2020_Simple_v7 (Autodesk Fusion 360 design; units mm, degrees)
Autodesk Fusion 360 part; units mm, degrees
sketch "Sketch1" plane through (0, 0, 0) normal (1, 0, 0) x (0, 1, 0)
  line L0 (4.6363, -9.9678) -> (4.6743, -9.9793) construction
  line L1 (-9.9374, 4.563) -> (-9.9187, 4.5279) construction
  line L2 (8.5, -10) -> (9.5, -10) construction
  line L3 (10, -9.5) -> (10, -8.5) construction
  line L4 (-9.8746, 4.4619) -> (-9.8494, 4.4312) construction
  line L5 (-9.9187, 4.5279) -> (-9.8977, 4.4942) construction
  line L6 (9.9987, -4.7917) -> (9.9948, -4.7522) construction
  line L7 (9.8977, -4.4942) -> (9.8746, -4.4619) construction
  arc A0 (-8.5414, 3.1214) -> (-8.2, 3.2628) centre (-8.4, 3.2628) ccw construction
  line L8 (10, -4.9) -> (9.9987, -4.7917) construction
  line L9 (-3.9, 2.8393) -> (-3.9, 0.1999) construction
  line L10 (-9.8977, 4.4942) -> (-9.8746, 4.4619) construction
  line L11 (-10, 4.8314) -> (-9.9987, 4.7917) construction
  line L12 (-9.8494, 4.4312) -> (-9.8222, 4.4022) construction
  line L13 (8.2, -5.5) -> (6.5607, -5.5) construction
  line L14 (-6.5607, 5.5) -> (-3.9, 2.8393) construction
  line L15 (5.5, -6.5607) -> (5.5, -8.2) construction
  line L16 (-3.9, 0.1999) -> (-3.7001, 0) construction
  line L17 (6.5607, -5.5) -> (3.9, -2.8393) construction
  line L18 (9.9987, 4.7917) -> (10, 4.9) construction
  line L19 (8.2, -3.2628) -> (8.2, -5.5) construction
  line L20 (-4.4942, 9.8977) -> (-4.5279, 9.9187) construction
  line L21 (9.9948, 4.7522) -> (9.9987, 4.7917) construction
  line L22 (9.8746, -4.4619) -> (9.8494, -4.4312) construction
  line L23 (9.9374, -4.563) -> (9.9187, -4.5279) construction
  line L24 (10, 8.5) -> (10, 9.5) construction
  line L25 (4.4312, -9.8494) -> (4.4619, -9.8746) construction
  line L26 (-8.2, 3.2628) -> (-8.2, 5.5) construction
  line L27 (4.4619, -9.8746) -> (4.4942, -9.8977) construction
  line L28 (-9.9883, 4.713) -> (-9.9793, 4.6743) construction
  line L29 (9.9883, 4.713) -> (9.9948, 4.7522) construction
  line L30 (-4.4312, 9.8494) -> (-4.4619, 9.8746) construction
  line L31 (10, 4.9) -> (10, 8.5) construction
  arc A1 (9.5, -10) -> (10, -9.5) centre (9.5, -9.5) ccw construction
  line L32 (9.9678, -4.6363) -> (9.9538, -4.5991) construction
  arc A2 (10, 9.5) -> (9.5, 10) centre (9.5, 9.5) ccw construction
  line L33 (4.5991, -9.9538) -> (4.6363, -9.9678) construction
  line L34 (-9.9538, 4.5991) -> (-9.9374, 4.563) construction
  line L35 (-9.9793, 4.6743) -> (-9.9678, 4.6363) construction
  line L36 (4.563, -9.9374) -> (4.5991, -9.9538) construction
  line L37 (1.1358, -3.9) -> (1.1358, -10) construction
  line L38 (-0.2048, -3.9) -> (0, -3.6952) construction
  line L39 (8.5414, 3.1214) -> (9.8222, 4.4022) construction
  line L40 (2.8393, 3.9) -> (0.207, 3.9) construction
  line L41 (0.207, 3.9) -> (0, 3.6952) construction
  line L42 (3.9, -0.1999) -> (3.7001, 0) construction
  line L43 (3.9, -2.8393) -> (3.9, -0.1999) construction
  line L44 (-3.9, -0.1999) -> (-3.9, -2.8393) construction
  line L45 (3.9, 0.1999) -> (3.9, 2.8393) construction
  line L46 (2.8393, 3.9) -> (0.207, 3.9) construction
  line L47 (0, 3.6952) -> (-0.2048, 3.9) construction
  line L48 (3.9, 2.8393) -> (6.5607, 5.5) construction
  line L49 (3.7001, 0) -> (3.9, 0.1999) construction
  line L50 (3.9, 0.1999) -> (3.9, 2.8393) construction
  arc A3 (-3.1214, -8.5414) -> (-3.2628, -8.2) centre (-3.2628, -8.4) ccw construction
  line L51 (0, -3.6952) -> (0.2048, -3.9) construction
  line L52 (-2.8393, -3.9) -> (-0.2048, -3.9) construction
  line L53 (3.9, -0.1999) -> (3.7001, 0) construction
  circle A4 centre (0, 0) radius 2.1 construction
  line L54 (3.7001, 0) -> (3.9, 0.1999) construction
  arc A5 (8.2, 3.2628) -> (8.5414, 3.1214) centre (8.4, 3.2628) ccw construction
  circle A6 centre (0, 0) radius 2.1 construction
  line L55 (5.5, 8.2) -> (5.5, 6.5607) construction
  line L56 (-4.6363, -9.9678) -> (-4.5991, -9.9538) construction
  line L57 (9.9883, 4.713) -> (9.9948, 4.7522) construction
  line L58 (3.2628, 8.2) -> (5.5, 8.2) construction
  line L59 (9.9538, 4.5991) -> (9.9678, 4.6363) construction
  arc A7 (8.2, 3.2628) -> (8.5414, 3.1214) centre (8.4, 3.2628) ccw construction
  line L60 (4.5991, 9.9538) -> (4.563, 9.9374) construction
  line L61 (-9.9538, -4.5991) -> (-9.9678, -4.6363) construction
  line L62 (-9.8977, -4.4942) -> (-9.9187, -4.5279) construction
  line L63 (-4.5279, -9.9187) -> (-4.4942, -9.8977) construction
  line L64 (0, 3.6952) -> (-0.2048, 3.9) construction
  arc A8 (3.1214, 8.5414) -> (3.2628, 8.2) centre (3.2628, 8.4) ccw construction
  line L65 (-9.8494, -4.4312) -> (-9.8746, -4.4619) construction
  line L66 (4.4942, 9.8977) -> (4.4619, 9.8746) construction
  line L67 (4.713, 9.9883) -> (4.6743, 9.9793) construction
  line L68 (-8.5, -10) -> (-4.8314, -10) construction
  line L69 (-9.5, -10) -> (-8.5, -10) construction
  line L70 (9.8222, 4.4022) -> (9.8494, 4.4312) construction
  line L71 (4.8314, 10) -> (4.7917, 9.9987) construction
  line L72 (-9.9948, -4.7522) -> (-9.9987, -4.7917) construction
  line L73 (4.6743, 9.9793) -> (4.6363, 9.9678) construction
  line L74 (5.5, 6.5607) -> (2.8393, 3.9) construction
  line L75 (4.4022, 9.8222) -> (3.1214, 8.5414) construction
  line L76 (-4.5991, -9.9538) -> (-4.563, -9.9374) construction
  line L77 (9.5, 10) -> (4.8314, 10) construction
  line L78 (0.207, 3.9) -> (0, 3.6952) construction
  line L79 (4.6363, 9.9678) -> (4.5991, 9.9538) construction
  line L80 (-9.9883, -4.713) -> (-9.9948, -4.7522) construction
  line L81 (4.7522, 9.9948) -> (4.713, 9.9883) construction
  line L82 (-4.4312, -9.8494) -> (-4.4022, -9.8222) construction
  line L83 (9.8746, 4.4619) -> (9.8977, 4.4942) construction
  line L84 (-8.2, -5.5) -> (-8.2, -3.2628) construction
  line L85 (10, 8.5) -> (10, 9.5) construction
  line L86 (3.2628, 8.2) -> (5.5, 8.2) construction
  arc A9 (3.1214, 8.5414) -> (3.2628, 8.2) centre (3.2628, 8.4) ccw construction
  arc A10 (10, 9.5) -> (9.5, 10) centre (9.5, 9.5) ccw construction
  line L87 (4.4619, 9.8746) -> (4.4312, 9.8494) construction
  line L88 (4.5279, 9.9187) -> (4.4942, 9.8977) construction
  line L89 (-4.6743, -9.9793) -> (-4.6363, -9.9678) construction
  line L90 (-4.7917, -9.9987) -> (-4.7522, -9.9948) construction
  line L91 (-9.9678, -4.6363) -> (-9.9793, -4.6743) construction
  line L92 (9.9793, 4.6743) -> (9.9883, 4.713) construction
  line L93 (-4.8314, -10) -> (-4.7917, -9.9987) construction
  line L94 (-9.9987, -4.7917) -> (-10, -4.8314) construction
  line L95 (5.5, 8.2) -> (5.5, 6.5607) construction
  line L96 (9.8977, 4.4942) -> (9.9187, 4.5279) construction
  arc A11 (-8.2, -3.2628) -> (-8.5414, -3.1214) centre (-8.4, -3.2628) ccw construction
  line L97 (-8.5414, -3.1214) -> (-9.8222, -4.4022) construction
  line L98 (4.563, 9.9374) -> (4.5279, 9.9187) construction
  line L99 (9.9374, 4.563) -> (9.9538, 4.5991) construction
  line L100 (9.8494, 4.4312) -> (9.8746, 4.4619) construction
  line L101 (-4.4942, -9.8977) -> (-4.4619, -9.8746) construction
  line L102 (-9.9187, -4.5279) -> (-9.9374, -4.563) construction
  arc A12 (-10, -9.5) -> (-9.5, -10) centre (-9.5, -9.5) ccw construction
  line L103 (-4.563, -9.9374) -> (-4.5279, -9.9187) construction
  line L104 (4.4022, 9.8222) -> (3.1214, 8.5414) construction
  line L105 (-6.5607, -5.5) -> (-8.2, -5.5) construction
  line L106 (10, 4.9) -> (10, 8.5) construction
  line L107 (3.9, 2.8393) -> (6.5607, 5.5) construction
  line L108 (4.4312, 9.8494) -> (4.4022, 9.8222) construction
  line L109 (9.9678, 4.6363) -> (9.9793, 4.6743) construction
  line L110 (-4.4619, -9.8746) -> (-4.4312, -9.8494) construction
  line L111 (-4.7522, -9.9948) -> (-4.713, -9.9883) construction
  line L112 (-10, -4.8314) -> (-10, -9.5) construction
  line L113 (4.5279, 9.9187) -> (4.4942, 9.8977) construction
  line L114 (9.9948, 4.7522) -> (9.9987, 4.7917) construction
  line L115 (4.7917, 9.9987) -> (4.7522, 9.9948) construction
  line L116 (4.563, 9.9374) -> (4.5279, 9.9187) construction
  line L117 (5.5, 6.5607) -> (2.8393, 3.9) construction
  line L118 (4.4619, 9.8746) -> (4.4312, 9.8494) construction
  line L119 (4.4942, 9.8977) -> (4.4619, 9.8746) construction
  line L120 (4.5991, 9.9538) -> (4.563, 9.9374) construction
  line L121 (-5.5, -8.2) -> (-5.5, -6.5607) construction
  line L122 (9.9987, 4.7917) -> (10, 4.9) construction
  line L123 (8.2, 5.5) -> (8.2, 3.2628) construction
  line L124 (4.4312, 9.8494) -> (4.4022, 9.8222) construction
  line L125 (-9.8746, -4.4619) -> (-9.8977, -4.4942) construction
  line L126 (-4.713, -9.9883) -> (-4.6743, -9.9793) construction
  line L127 (9.9187, 4.5279) -> (9.9374, 4.563) construction
  line L128 (6.5607, 5.5) -> (8.2, 5.5) construction
  line L129 (-9.9793, -4.6743) -> (-9.9883, -4.713) construction
  line L130 (-5.5, -6.5607) -> (-2.8393, -3.9) construction
  line L131 (8.5414, 3.1214) -> (9.8222, 4.4022) construction
  line L132 (-3.9, -2.8393) -> (-6.5607, -5.5) construction
  line L133 (4.713, 9.9883) -> (4.6743, 9.9793) construction
  line L134 (4.7917, 9.9987) -> (4.7522, 9.9948) construction
  line L135 (-4.4022, -9.8222) -> (-3.1214, -8.5414) construction
  line L136 (-9.9987, 4.7917) -> (-9.9948, 4.7522) construction
  line L137 (4.6363, 9.9678) -> (4.5991, 9.9538) construction
  line L138 (4.8314, 10) -> (4.7917, 9.9987) construction
  line L139 (-9.9948, 4.7522) -> (-9.9883, 4.713) construction
  line L140 (4.6743, 9.9793) -> (4.6363, 9.9678) construction
  line L141 (-8.2, 5.5) -> (-6.5607, 5.5) construction
  line L142 (-3.7001, 0) -> (-3.9, -0.1999) construction
  line L143 (-9.9678, 4.6363) -> (-9.9538, 4.5991) construction
  line L144 (-9.8222, 4.4022) -> (-8.5414, 3.1214) construction
  line L145 (-9.9374, -4.563) -> (-9.9538, -4.5991) construction
  line L146 (-9.8222, -4.4022) -> (-9.8494, -4.4312) construction
  line L147 (4.7522, 9.9948) -> (4.713, 9.9883) construction
  line L148 (-3.2628, -8.2) -> (-5.5, -8.2) construction
  line L149 (4.4619, -9.8746) -> (4.4942, -9.8977) construction
  line L150 (-9.9948, 4.7522) -> (-9.9883, 4.713) construction
  line L151 (4.5279, -9.9187) -> (4.563, -9.9374) construction
  line L152 (-9.9793, 4.6743) -> (-9.9678, 4.6363) construction
  line L153 (-9.9883, 4.713) -> (-9.9793, 4.6743) construction
  line L154 (4.4312, -9.8494) -> (4.4619, -9.8746) construction
  line L155 (-9.8977, 4.4942) -> (-9.8746, 4.4619) construction
  line L156 (4.7522, -9.9948) -> (4.7917, -9.9987) construction
  line L157 (4.713, -9.9883) -> (4.7522, -9.9948) construction
  line L158 (4.4942, -9.8977) -> (4.5279, -9.9187) construction
  line L159 (4.5991, -9.9538) -> (4.6363, -9.9678) construction
  line L160 (-9.9187, 4.5279) -> (-9.8977, 4.4942) construction
  line L161 (4.6743, -9.9793) -> (4.713, -9.9883) construction
  line L162 (4.563, -9.9374) -> (4.5991, -9.9538) construction
  line L163 (-9.9678, 4.6363) -> (-9.9538, 4.5991) construction
  line L164 (-9.9538, 4.5991) -> (-9.9374, 4.563) construction
  line L165 (-9.9374, 4.563) -> (-9.9187, 4.5279) construction
  line L166 (-9.8746, 4.4619) -> (-9.8494, 4.4312) construction
  line L167 (4.6363, -9.9678) -> (4.6743, -9.9793) construction
  line L168 (-4.7522, 9.9948) -> (-4.7917, 9.9987) construction
  line L169 (9.8494, 4.4312) -> (9.8746, 4.4619) construction
  line L170 (4.5279, -9.9187) -> (4.563, -9.9374) construction
  line L171 (-4.5991, 9.9538) -> (-4.6363, 9.9678) construction
  line L172 (9.9538, -4.5991) -> (9.9374, -4.563) construction
  line L173 (-10, 9.5) -> (-10, 8.5) construction
  line L174 (9.8977, 4.4942) -> (9.9187, 4.5279) construction
  line L175 (4.8314, -10) -> (8.5, -10) construction
  line L176 (9.8746, 4.4619) -> (9.8977, 4.4942) construction
  line L177 (4.7917, -9.9987) -> (4.8314, -10) construction
  line L178 (-5.5, 8.2) -> (-3.2628, 8.2) construction
  line L179 (9.9793, 4.6743) -> (9.9883, 4.713) construction
  line L180 (4.713, -9.9883) -> (4.7522, -9.9948) construction
  arc A13 (-9.5, 10) -> (-10, 9.5) centre (-9.5, 9.5) ccw construction
  line L181 (2.8393, -3.9) -> (5.5, -6.5607) construction
  line L182 (9.8494, -4.4312) -> (9.8222, -4.4022) construction
  line L183 (9.9187, -4.5279) -> (9.8977, -4.4942) construction
  line L184 (10, -8.5) -> (10, -4.9) construction
  line L185 (-4.563, 9.9374) -> (-4.5991, 9.9538) construction
  line L186 (-4.6743, 9.9793) -> (-4.713, 9.9883) construction
  line L187 (-5.5, 6.5607) -> (-5.5, 8.2) construction
  line L188 (-4.8314, 10) -> (-8.5, 10) construction
  line L189 (9.9374, 4.563) -> (9.9538, 4.5991) construction
  line L190 (-8.5, 10) -> (-9.5, 10) construction
  line L191 (-4.7917, 9.9987) -> (-4.8314, 10) construction
  line L192 (-4.5279, 9.9187) -> (-4.563, 9.9374) construction
  line L193 (9.9538, 4.5991) -> (9.9678, 4.6363) construction
  line L194 (-4.6363, 9.9678) -> (-4.6743, 9.9793) construction
  line L195 (4.7522, -9.9948) -> (4.7917, -9.9987) construction
  line L196 (-3.1214, 8.5414) -> (-4.4022, 9.8222) construction
  line L197 (5.5, -8.2) -> (3.2628, -8.2) construction
  line L198 (9.9793, -4.6743) -> (9.9678, -4.6363) construction
  line L199 (4.6743, -9.9793) -> (4.713, -9.9883) construction
  line L200 (9.9187, 4.5279) -> (9.9374, 4.563) construction
  line L201 (9.9948, -4.7522) -> (9.9883, -4.713) construction
  line L202 (9.8222, -4.4022) -> (8.5414, -3.1214) construction
  line L203 (-4.713, 9.9883) -> (-4.7522, 9.9948) construction
  line L204 (9.9678, 4.6363) -> (9.9793, 4.6743) construction
  line L205 (9.9883, -4.713) -> (9.9793, -4.6743) construction
  arc A14 (-3.2628, 8.2) -> (-3.1214, 8.5414) centre (-3.2628, 8.4) ccw construction
  line L206 (4.4022, -9.8222) -> (4.4312, -9.8494) construction
  arc A15 (8.5414, -3.1214) -> (8.2, -3.2628) centre (8.4, -3.2628) ccw construction
  arc A16 (3.2628, -8.2) -> (3.1214, -8.5414) centre (3.2628, -8.4) ccw construction
  line L207 (9.8222, 4.4022) -> (9.8494, 4.4312) construction
  line L208 (-3.9, 0.1999) -> (-3.7001, 0) construction
  line L209 (-0.2048, 3.9) -> (-2.8393, 3.9) construction
  line L210 (8.2, 5.5) -> (8.2, 3.2628) construction
  line L211 (6.6657, -10) -> (-6.6657, -10) construction
  line L212 (-3.7001, 0) -> (-3.9, -0.1999) construction
  line L213 (4.4942, -9.8977) -> (4.5279, -9.9187) construction
  line L214 (0.2048, -3.9) -> (2.8393, -3.9) construction
  line L215 (-10, 8.5) -> (-10, 4.8314) construction
  line L216 (2.8393, -3.9) -> (5.5, -6.5607) construction
  line L217 (-2.8393, 3.9) -> (-5.5, 6.5607) construction
  line L218 (-0.2048, -3.9) -> (0, -3.6952) construction
  line L219 (5.5, -6.5607) -> (5.5, -8.2) construction
  line L220 (3.9, -2.8393) -> (3.9, -0.1999) construction
  line L221 (-4.4022, 9.8222) -> (-4.4312, 9.8494) construction
  line L222 (-0.2048, 3.9) -> (-2.8393, 3.9) construction
  line L223 (-4.4619, 9.8746) -> (-4.4942, 9.8977) construction
  line L224 (0.2048, -3.9) -> (2.8393, -3.9) construction
  line L225 (3.1214, -8.5414) -> (4.4022, -9.8222) construction
  line L226 (9.5, 10) -> (4.8314, 10) construction
  line L227 (0, -3.6952) -> (0.2048, -3.9) construction
  line L228 (6.5607, 5.5) -> (8.2, 5.5) construction
  line L229 (-2.8393, 3.9) -> (-5.5, 6.5607) construction
  line L230 (-3.9, 2.8393) -> (-3.9, 0.1999) construction
  line L231 (-6.5607, 5.5) -> (-3.9, 2.8393) construction
  arc A17 (-8.5414, 3.1214) -> (-8.2, 3.2628) centre (-8.4, 3.2628) ccw construction
  arc A18 (3.2628, -8.2) -> (3.1214, -8.5414) centre (3.2628, -8.4) ccw construction
  line L232 (-9.8222, 4.4022) -> (-8.5414, 3.1214) construction
  line L233 (-9.8494, 4.4312) -> (-9.8222, 4.4022) construction
  line L234 (-8.2, 5.5) -> (-6.5607, 5.5) construction
  line L235 (4.7917, -9.9987) -> (4.8314, -10) construction
  line L236 (8.5, -10) -> (9.5, -10) construction
  line L237 (4.8314, -10) -> (8.5, -10) construction
  line L238 (-9.5, -10) -> (-8.5, -10) construction
  line L239 (-5.5, -8.2) -> (-5.5, -6.5607) construction
  line L240 (-4.4619, -9.8746) -> (-4.4312, -9.8494) construction
  line L241 (-4.6363, -9.9678) -> (-4.5991, -9.9538) construction
  line L242 (-4.563, -9.9374) -> (-4.5279, -9.9187) construction
  line L243 (-4.7522, -9.9948) -> (-4.713, -9.9883) construction
  line L244 (-8.2, -5.5) -> (-8.2, -3.2628) construction
  arc A19 (-10, -9.5) -> (-9.5, -10) centre (-9.5, -9.5) ccw construction
  line L245 (-4.6743, -9.9793) -> (-4.6363, -9.9678) construction
  line L246 (-4.713, -9.9883) -> (-4.6743, -9.9793) construction
  line L247 (-4.5279, -9.9187) -> (-4.4942, -9.8977) construction
  line L248 (-4.5991, -9.9538) -> (-4.563, -9.9374) construction
  line L249 (-5.5, 8.2) -> (-3.2628, 8.2) construction
  line L250 (6.5607, -5.5) -> (3.9, -2.8393) construction
  line L251 (-3.2628, -8.2) -> (-5.5, -8.2) construction
  line L252 (-4.8314, -10) -> (-4.7917, -9.9987) construction
  line L253 (-4.8314, 10) -> (-8.5, 10) construction
  line L254 (8.2, -3.2628) -> (8.2, -5.5) construction
  line L255 (-4.4312, -9.8494) -> (-4.4022, -9.8222) construction
  line L256 (10, -8.5) -> (10, -4.9) construction
  line L257 (-4.4942, -9.8977) -> (-4.4619, -9.8746) construction
  line L258 (-10, -4.8314) -> (-10, -9.5) construction
  line L259 (-8.5, -10) -> (-4.8314, -10) construction
  line L260 (-4.4022, -9.8222) -> (-3.1214, -8.5414) construction
  arc A20 (-3.1214, -8.5414) -> (-3.2628, -8.2) centre (-3.2628, -8.4) ccw construction
  line L261 (-4.7917, -9.9987) -> (-4.7522, -9.9948) construction
  arc A21 (8.5414, -3.1214) -> (8.2, -3.2628) centre (8.4, -3.2628) ccw construction
  line L262 (-6.5607, -5.5) -> (-8.2, -5.5) construction
  line L263 (-3.9, -2.8393) -> (-6.5607, -5.5) construction
  line L264 (-8.2, 3.2628) -> (-8.2, 5.5) construction
  line L265 (4.4022, -9.8222) -> (4.4312, -9.8494) construction
  line L266 (-10, 4.8314) -> (-9.9987, 4.7917) construction
  line L267 (5.5, -8.2) -> (3.2628, -8.2) construction
  line L268 (-10, 8.5) -> (-10, 4.8314) construction
  line L269 (-9.9987, 4.7917) -> (-9.9948, 4.7522) construction
  line L270 (-2.8393, -3.9) -> (-0.2048, -3.9) construction
  line L271 (3.1214, -8.5414) -> (4.4022, -9.8222) construction
  line L272 (-5.5, -6.5607) -> (-2.8393, -3.9) construction
  arc A22 (-3.2628, 8.2) -> (-3.1214, 8.5414) centre (-3.2628, 8.4) ccw construction
  line L273 (-3.9, -0.1999) -> (-3.9, -2.8393) construction
  line L274 (-4.7917, 9.9987) -> (-4.8314, 10) construction
  line L275 (9.8222, -4.4022) -> (8.5414, -3.1214) construction
  line L276 (-9.9678, -4.6363) -> (-9.9793, -4.6743) construction
  line L277 (9.9793, -4.6743) -> (9.9678, -4.6363) construction
  line L278 (-4.6363, 9.9678) -> (-4.6743, 9.9793) construction
  line L279 (-4.7522, 9.9948) -> (-4.7917, 9.9987) construction
  line L280 (-9.9374, -4.563) -> (-9.9538, -4.5991) construction
  line L281 (9.9987, -4.7917) -> (9.9948, -4.7522) construction
  line L282 (-4.5991, 9.9538) -> (-4.6363, 9.9678) construction
  line L283 (-4.713, 9.9883) -> (-4.7522, 9.9948) construction
  line L284 (-4.6743, 9.9793) -> (-4.713, 9.9883) construction
  line L285 (-9.9948, -4.7522) -> (-9.9987, -4.7917) construction
  line L286 (-9.9883, -4.713) -> (-9.9948, -4.7522) construction
  line L287 (-4.4619, 9.8746) -> (-4.4942, 9.8977) construction
  line L288 (9.8977, -4.4942) -> (9.8746, -4.4619) construction
  line L289 (9.9187, -4.5279) -> (9.8977, -4.4942) construction
  line L290 (-9.9987, -4.7917) -> (-10, -4.8314) construction
  line L291 (-4.4942, 9.8977) -> (-4.5279, 9.9187) construction
  line L292 (-4.5279, 9.9187) -> (-4.563, 9.9374) construction
  line L293 (-4.4312, 9.8494) -> (-4.4619, 9.8746) construction
  line L294 (-4.563, 9.9374) -> (-4.5991, 9.9538) construction
  line L295 (-4.4022, 9.8222) -> (-4.4312, 9.8494) construction
  line L296 (9.9374, -4.563) -> (9.9187, -4.5279) construction
  arc A23 (-8.2, -3.2628) -> (-8.5414, -3.1214) centre (-8.4, -3.2628) ccw construction
  line L297 (9.9538, -4.5991) -> (9.9374, -4.563) construction
  line L298 (9.8494, -4.4312) -> (9.8222, -4.4022) construction
  line L299 (9.8746, -4.4619) -> (9.8494, -4.4312) construction
  line L300 (9.9678, -4.6363) -> (9.9538, -4.5991) construction
  line L301 (-9.9793, -4.6743) -> (-9.9883, -4.713) construction
  line L302 (-9.9538, -4.5991) -> (-9.9678, -4.6363) construction
  line L303 (-3.1214, 8.5414) -> (-4.4022, 9.8222) construction
  line L304 (9.9883, -4.713) -> (9.9793, -4.6743) construction
  line L305 (9.9948, -4.7522) -> (9.9883, -4.713) construction
  line L306 (-9.8222, -4.4022) -> (-9.8494, -4.4312) construction
  line L307 (8.2, -5.5) -> (6.5607, -5.5) construction
  arc A24 (9.5, -10) -> (10, -9.5) centre (9.5, -9.5) ccw construction
  line L308 (-8.5414, -3.1214) -> (-9.8222, -4.4022) construction
  line L309 (10, -9.5) -> (10, -8.5) construction
  line L310 (10, -4.9) -> (9.9987, -4.7917) construction
  line L311 (-9.8977, -4.4942) -> (-9.9187, -4.5279) construction
  arc A25 (-9.5, 10) -> (-10, 9.5) centre (-9.5, 9.5) ccw construction
  line L312 (-9.8494, -4.4312) -> (-9.8746, -4.4619) construction
  line L313 (-9.9187, -4.5279) -> (-9.9374, -4.563) construction
  line L314 (-8.5, 10) -> (-9.5, 10) construction
  line L315 (-10, 9.5) -> (-10, 8.5) construction
  line L316 (-5.5, 6.5607) -> (-5.5, 8.2) construction
  line L317 (-9.8746, -4.4619) -> (-9.8977, -4.4942) construction
  line L318 (3.9, 2.8393) -> (3.9, -2.8393)
  line L319 (3.9, -2.8393) -> (6.5607, -5.5)
  line L320 (6.5607, -5.5) -> (8.2, -5.5)
  line L321 (8.2, -5.5) -> (8.2, -3.2628)
  line L322 (8.5414, -3.1214) -> (9.8222, -4.4022)
  arc A26 (8.5414, -3.1214) -> (8.2, -3.2628) centre (8.4, -3.2628) ccw
  line L323 (10, -9.5) -> (9.9987, -4.7917)
  line L324 (9.5, -10) -> (4.8314, -10)
  line L325 (3.1214, -8.5414) -> (4.4022, -9.8222)
  line L326 (3.2628, -8.2) -> (5.5, -8.2)
  line L327 (5.5, -8.2) -> (5.5, -6.5607)
  arc A27 (9.5, -10) -> (10, -9.5) centre (9.5, -9.5) ccw
  arc A28 (9.9987, -4.7917) -> (9.8222, -4.4022) centre (9.3929, -4.8314) ccw
  line L328 (5.5, -6.5607) -> (2.8393, -3.9)
  line L329 (2.8393, -3.9) -> (-2.8393, -3.9)
  line L330 (-2.8393, -3.9) -> (-5.5, -6.5607)
  line L331 (-5.5, -6.5607) -> (-5.5, -8.2)
  line L332 (-5.5, -8.2) -> (-3.2628, -8.2)
  line L333 (-3.1214, -8.5414) -> (-4.2336, -9.6536)
  line L334 (-9.5, -10) -> (-4.8314, -10)
  line L335 (-10, -9.5) -> (-10, -4.8314)
  line L336 (-9.8222, -4.4022) -> (-8.5414, -3.1214)
  line L337 (-8.2, -3.2628) -> (-8.2, -5.5)
  line L338 (-8.2, -5.5) -> (-6.5607, -5.5)
  line L339 (-6.5607, -5.5) -> (-3.9, -2.8393)
  line L340 (-3.9, -2.8393) -> (-3.9, 2.8393)
  line L341 (-3.9, 2.8393) -> (-6.5607, 5.5)
  line L342 (-6.5607, 5.5) -> (-8.2, 5.5)
  line L343 (-8.2, 5.5) -> (-8.2, 3.2628)
  line L344 (-8.5414, 3.1214) -> (-9.8222, 4.4022)
  line L345 (-10, 9.5) -> (-10, 4.8314)
  line L346 (-9.5, 10) -> (-4.8314, 10)
  line L347 (-5.5, 8.2) -> (-3.2628, 8.2)
  line L348 (-3.1214, 8.5414) -> (-4.4022, 9.8222)
  line L349 (-5.5, 8.2) -> (-5.5, 6.5607)
  line L350 (-5.5, 6.5607) -> (-2.8393, 3.9)
  line L351 (-2.8393, 3.9) -> (2.8393, 3.9)
  line L352 (2.8393, 3.9) -> (5.5, 6.5607)
  line L353 (5.5, 6.5607) -> (5.5, 8.2)
  line L354 (5.5, 8.2) -> (3.2628, 8.2)
  line L355 (3.1214, 8.5414) -> (4.4312, 9.8494)
  line L356 (3.9, 2.8393) -> (6.5607, 5.5)
  line L357 (6.5607, 5.5) -> (8.2, 5.5)
  line L358 (8.2, 5.5) -> (8.2, 3.2628)
  line L359 (8.5414, 3.1214) -> (9.8494, 4.4312)
  line L360 (10, 4.9) -> (10, 9.5)
  line L361 (9.5, 10) -> (4.8314, 10)
  arc A29 (8.2, 3.2628) -> (8.5414, 3.1214) centre (8.4, 3.2628) ccw
  arc A30 (9.8494, 4.4312) -> (10, 4.9) centre (9.3734, 4.8428) ccw
  arc A31 (10, 9.5) -> (9.5, 10) centre (9.5, 9.5) ccw
  arc A32 (4.8314, 10) -> (4.4312, 9.8494) centre (4.8314, 9.3929) ccw
  arc A33 (3.1214, 8.5414) -> (3.2628, 8.2) centre (3.2628, 8.4) ccw
  arc A34 (-3.2628, 8.2) -> (-3.1214, 8.5414) centre (-3.2628, 8.4) ccw
  arc A35 (-4.4022, 9.8222) -> (-4.8314, 10) centre (-4.8314, 9.3929) ccw
  arc A36 (-9.5, 10) -> (-10, 9.5) centre (-9.5, 9.5) ccw
  arc A37 (-10, 4.8314) -> (-9.8222, 4.4022) centre (-9.3929, 4.8314) ccw
  arc A38 (-8.5414, 3.1214) -> (-8.2, 3.2628) centre (-8.4, 3.2628) ccw
  arc A39 (-8.2, -3.2628) -> (-8.5414, -3.1214) centre (-8.4, -3.2628) ccw
  arc A40 (-9.8222, -4.4022) -> (-10, -4.8314) centre (-9.3929, -4.8314) ccw
  arc A41 (-10, -9.5) -> (-9.5, -10) centre (-9.5, -9.5) ccw
  arc A42 (-4.8314, -10) -> (-4.2336, -9.6536) centre (-4.8837, -9.2207) ccw
  arc A43 (-3.1214, -8.5414) -> (-3.2628, -8.2) centre (-3.2628, -8.4) ccw
  arc A44 (3.2628, -8.2) -> (3.1214, -8.5414) centre (3.2628, -8.4) ccw
  arc A45 (4.4022, -9.8222) -> (4.8314, -10) centre (4.8314, -9.3929) ccw
  circle A46 centre (0, 0) radius 2.1
  constraint midpoint L211.start L175
  constraint midpoint L211.end L68
  constraint coincident L37.start L214
  constraint coincident L37.end L211
  constraint perpendicular L37 L211
  constraint parallel L220 L318
  constraint parallel L17 L319
  constraint parallel L13 L320
  constraint tangent A15 L321
  constraint tangent A21 L322
  constraint tangent L275 A26
  constraint tangent L19 A26
  constraint tangent A16 L325
  constraint tangent A16 L326
  constraint parallel L219 L327
  constraint coincident L32.end A28
  constraint parallel L181 L328
  constraint parallel L270 L329
  constraint parallel L272 L330
  constraint parallel L239 L331
  constraint tangent A20 L332
  constraint coincident L260 L333.end
  constraint tangent A3 L333
  constraint parallel L260 L333
  constraint horizontal L334
  constraint coincident L93 L68.end
  constraint tangent A19 L334
  constraint parallel L258 L335
  constraint tangent A23 L336
  constraint tangent A11 L337
  constraint parallel L105 L338
  constraint parallel L263 L339
  constraint parallel L230 L340
  constraint parallel L14 L341
  constraint parallel L141 L342
  constraint tangent A17 L343
  constraint tangent A0 L344
  constraint coincident L173.start L315
  constraint tangent A14 L347
  constraint tangent A22 L348
  constraint parallel L316 L349
  constraint parallel L217 L350
  constraint parallel L74 L352
  constraint parallel L55 L353
  constraint tangent A8 L354
  constraint parallel L107 L356
  constraint parallel L228 L357
  constraint tangent A5 L358
  constraint tangent A10 L360
  constraint parallel L77 L361
  constraint coincident L59.end A30
  constraint coincident L60.start A32
  constraint coincident L185.start A35
  constraint coincident L1.end A37
  constraint coincident L61.start A40
  constraint coincident L63.end A42
  constraint coincident L0.start A45
  constraint concentric A6 A46
extrude "Extrude1" add sketch "Sketch1" along normal blind 50
sketch "Sketch2" plane through (0, 0, 0) normal (-1, 0, 0) x (0, -1, 0)
  circle A0 centre (0, 0) radius 2.1
  arc A1 (-3.1214, -8.5414) -> (-3.2628, -8.2) centre (-3.2628, -8.4) ccw
  line L0 (-3.2628, -8.2) -> (-5.5, -8.2)
  line L1 (-5.5, -8.2) -> (-5.5, -6.5607)
  line L2 (-5.5, -6.5607) -> (-2.8393, -3.9)
  line L3 (-2.8393, -3.9) -> (2.8393, -3.9)
  line L4 (2.8393, -3.9) -> (5.5, -6.5607)
  line L5 (5.5, -6.5607) -> (5.5, -8.2)
  line L6 (5.5, -8.2) -> (3.2628, -8.2)
  arc A2 (3.2628, -8.2) -> (3.1214, -8.5414) centre (3.2628, -8.4) ccw
  line L7 (3.1214, -8.5414) -> (4.2336, -9.6536)
  arc A3 (4.2336, -9.6536) -> (4.8314, -10) centre (4.8837, -9.2207) ccw
  line L8 (4.8314, -10) -> (9.5, -10)
  arc A4 (9.5, -10) -> (10, -9.5) centre (9.5, -9.5) ccw
  line L9 (10, -9.5) -> (10, -4.8314)
  arc A5 (10, -4.8314) -> (9.8222, -4.4022) centre (9.3929, -4.8314) ccw
  line L10 (9.8222, -4.4022) -> (8.5414, -3.1214)
  arc A6 (8.5414, -3.1214) -> (8.2, -3.2628) centre (8.4, -3.2628) ccw
  line L11 (8.2, -3.2628) -> (8.2, -5.5)
  line L12 (8.2, -5.5) -> (6.5607, -5.5)
  line L13 (6.5607, -5.5) -> (3.9, -2.8393)
  line L14 (3.9, -2.8393) -> (3.9, 2.8393)
  line L15 (3.9, 2.8393) -> (6.5607, 5.5)
  line L16 (6.5607, 5.5) -> (8.2, 5.5)
  line L17 (8.2, 5.5) -> (8.2, 3.2628)
  arc A7 (8.2, 3.2628) -> (8.5414, 3.1214) centre (8.4, 3.2628) ccw
  line L18 (8.5414, 3.1214) -> (9.8222, 4.4022)
  arc A8 (9.8222, 4.4022) -> (10, 4.8314) centre (9.3929, 4.8314) ccw
  line L19 (10, 4.8314) -> (10, 9.5)
  arc A9 (10, 9.5) -> (9.5, 10) centre (9.5, 9.5) ccw
  line L20 (9.5, 10) -> (4.8314, 10)
  arc A10 (4.8314, 10) -> (4.4022, 9.8222) centre (4.8314, 9.3929) ccw
  line L21 (4.4022, 9.8222) -> (3.1214, 8.5414)
  arc A11 (3.1214, 8.5414) -> (3.2628, 8.2) centre (3.2628, 8.4) ccw
  line L22 (3.2628, 8.2) -> (5.5, 8.2)
  line L23 (5.5, 8.2) -> (5.5, 6.5607)
  line L24 (5.5, 6.5607) -> (2.8393, 3.9)
  line L25 (2.8393, 3.9) -> (-2.8393, 3.9)
  line L26 (-2.8393, 3.9) -> (-5.5, 6.5607)
  line L27 (-5.5, 6.5607) -> (-5.5, 8.2)
  line L28 (-5.5, 8.2) -> (-3.2628, 8.2)
  arc A12 (-3.2628, 8.2) -> (-3.1214, 8.5414) centre (-3.2628, 8.4) ccw
  line L29 (-3.1214, 8.5414) -> (-4.4312, 9.8494)
  arc A13 (-4.4312, 9.8494) -> (-4.8314, 10) centre (-4.8314, 9.3929) ccw
  line L30 (-4.8314, 10) -> (-9.5, 10)
  arc A14 (-9.5, 10) -> (-10, 9.5) centre (-9.5, 9.5) ccw
  line L31 (-10, 9.5) -> (-10, 4.9)
  arc A15 (-10, 4.9) -> (-9.8494, 4.4312) centre (-9.3734, 4.8428) ccw
  line L32 (-9.8494, 4.4312) -> (-8.5414, 3.1214)
  arc A16 (-8.5414, 3.1214) -> (-8.2, 3.2628) centre (-8.4, 3.2628) ccw
  line L33 (-8.2, 3.2628) -> (-8.2, 5.5)
  line L34 (-8.2, 5.5) -> (-6.5607, 5.5)
  line L35 (-6.5607, 5.5) -> (-3.9, 2.8393)
  line L36 (-3.9, 2.8393) -> (-3.9, -2.8393)
  line L37 (-3.9, -2.8393) -> (-6.5607, -5.5)
  line L38 (-6.5607, -5.5) -> (-8.2, -5.5)
  line L39 (-8.2, -5.5) -> (-8.2, -3.2628)
  arc A17 (-8.2, -3.2628) -> (-8.5414, -3.1214) centre (-8.4, -3.2628) ccw
  line L40 (-8.5414, -3.1214) -> (-9.8222, -4.4022)
  arc A18 (-9.8222, -4.4022) -> (-9.9987, -4.7917) centre (-9.3929, -4.8314) ccw
  line L41 (-9.9987, -4.7917) -> (-10, -9.5)
  arc A19 (-10, -9.5) -> (-9.5, -10) centre (-9.5, -9.5) ccw
  line L42 (-9.5, -10) -> (-4.8314, -10)
  arc A20 (-4.8314, -10) -> (-4.4022, -9.8222) centre (-4.8314, -9.3929) ccw
  line L43 (-4.4022, -9.8222) -> (-3.1214, -8.5414)
  line L44 (-5.8557, 10) -> (6.4454, 10) construction
  constraint coincident L30 L44.start
  constraint coincident L20 L44.end
